Autodesk Inventor part; units mm, degrees
(part 2 of 3)
  spline S67 degree 3 poles (13.389509, -18.082427) (13.389509, -18.082427) (13.389509, -18.082427) (13.389509, -18.082427) (13.389509, -18.082427) (13.389509, -18.082427) (13.389509, -18.082427) (13.389509, -18.082427) (13.389509, -18.082427) (13.389509, -18.082427) (13.389509, -18.082427) (13.389509, -18.082427) (13.389509, -18.082427) (13.389509, -18.082427) (13.389509, -18.082427) (13.389449, -18.0824) (13.38145, -18.07871) (13.356188, -18.066962) (13.343085, -18.060852) (13.309671, -18.045163) (13.288775, -18.035295) (13.232029, -18.008233) (13.193942, -17.989858) (13.106898, -17.947135) (13.057393, -17.922403) (13.008015, -17.897214) knots 0 0 0 0 0.00003245 0.00003245 0.0000697 0.0000697 0.00012943 0.00012943 0.00021582 0.00021582 0.0003445 0.0003445 0.00053795 0.00053795 0.00077231 0.00077231 0.2100469 0.2100469 0.34914837 0.34914837 0.50737768 0.50737768 0.73605088 0.73605088 1 1 1 1
  arc A96 (13.389509, -18.082427) -> (14.254505, -17.40868) centre (0.000012, -0.000078) ccw
  arc A97 (13.008015, -17.897214) -> (14.168315, -16.993453) centre (0.000012, -0.000078) ccw
  arc A98 (13.008015, -17.897214) -> (14.168315, -16.993453) centre (0.000012, -0.000078) ccw
  spline S68 degree 3 poles (13.008015, -17.897214) (12.958136, -17.87177) (12.820927, -17.80036) (12.598988, -17.678088) (12.344986, -17.525914) (12.096924, -17.364239) (11.855202, -17.193219) (11.620622, -17.01253) (11.392126, -16.824355) (11.190356, -16.632755) (11.076365, -16.494814) (11.025839, -16.432401) knots 0 0 0 0 0.06771151 0.18704119 0.30636988 0.42569807 0.54502619 0.66435448 0.78368001 0.9029743 1 1 1 1
  spline S69 degree 3 poles (9.627578, -17.288804) (9.660216, -17.362174) (9.731294, -17.526398) (9.810284, -17.793198) (9.874079, -18.082249) (9.928439, -18.373318) (9.970943, -18.666356) (10.002239, -18.960794) (10.022375, -19.256206) (10.030442, -19.50947) (10.031705, -19.664143) (10.031705, -19.720138) knots 0 0 0 0 0.0970257 0.21631999 0.33564552 0.45497381 0.57430193 0.69363012 0.81295881 0.93228849 1 1 1 1
  spline S70 degree 3 poles (10.031705, -19.720138) (10.031705, -19.751925) (10.031556, -19.783696) (10.030978, -19.847374) (10.030538, -19.879187) (10.029238, -19.951858) (10.028283, -19.991171) (10.026684, -20.047685) (10.02605, -20.067721) (10.024929, -20.101167) (10.024444, -20.11462) (10.023769, -20.132892) (10.023548, -20.13864) (10.023433, -20.141656) (10.023401, -20.142482) (10.023369, -20.143307) (10.023337, -20.144133) knots 0 0 0 0 0.15652251 0.15652251 0.32009373 0.32009373 0.5482425 0.5482425 0.69838233 0.69838233 0.84400588 0.84400588 0.96648092 0.96648092 0.96648092 1 1 1 1
  arc A99 (9.030105, -20.608508) -> (10.023337, -20.144133) centre (0.000012, -0.000078) ccw
  arc A100 (8.69939, -20.343048) -> (10.031705, -19.720138) centre (0.000012, -0.000078) ccw
  arc A101 (8.69939, -20.343048) -> (10.031705, -19.720138) centre (0.000012, -0.000078) ccw
  spline S71 degree 3 poles (9.030105, -20.608508) (9.029452, -20.608004) (9.028799, -20.6075) (9.028146, -20.606995) (9.025218, -20.604734) (9.019043, -20.599964) (9.00106, -20.586016) (8.989646, -20.577144) (8.960561, -20.554413) (8.942385, -20.540143) (8.893084, -20.501131) (8.86004, -20.474743) (8.784685, -20.413721) (8.741925, -20.378593) (8.69939, -20.343048) knots 0 0 0 0 0.03353482 0.03353482 0.03353482 0.18383321 0.18383321 0.32755059 0.32755059 0.49103057 0.49103057 0.72729202 0.72729202 1 1 1 1
  arc A102 (7.092863, -18.473885) -> (6.374109, -18.179512) centre (6.56767, -18.731562) ccw
  spline S72 degree 3 poles (8.69939, -20.343048) (8.656423, -20.307143) (8.538545, -20.206992) (8.349378, -20.038399) (8.135606, -19.833519) (7.92974, -19.6207) (7.732134, -19.400179) (7.543642, -19.171822) (7.362748, -18.937519) (7.208672, -18.705825) (7.128233, -18.545977) (7.092863, -18.473885) knots 0 0 0 0 0.06771151 0.18704119 0.30636988 0.42569807 0.54502619 0.66435448 0.78368001 0.9029743 1 1 1 1
  arc A103 (5.932935, -18.328236) -> (6.374109, -18.179512) centre (0.000012, -0.000078) ccw
  arc A104 (5.932935, -18.328236) -> (5.539091, -18.997675) centre (6.113099, -18.884802) ccw
  spline S73 degree 3 poles (1.172852, -19.753927) (1.170424, -19.834191) (1.163209, -20.012992) (1.118616, -20.287643) (1.050679, -20.575748) (0.973366, -20.861578) (0.884515, -21.144038) (0.784961, -21.422896) (0.674928, -21.69779) (0.57231, -21.929473) (0.506337, -22.069377) (0.482042, -22.119826) knots 0 0 0 0 0.0970257 0.21631999 0.33564552 0.45497381 0.57430193 0.69363012 0.81295881 0.93228849 1 1 1 1
  arc A105 (1.705785, -19.18891) -> (1.172852, -19.753927) centre (1.757584, -19.771613) ccw
  arc A106 (1.705785, -19.18891) -> (2.168992, -19.142086) centre (0.000012, -0.000078) ccw
  arc A107 (2.804221, -19.589016) -> (2.168992, -19.142086) centre (2.234857, -19.723366) ccw
  spline S74 degree 3 poles (3.954541, -21.768801) (3.920641, -21.724235) (3.828004, -21.600365) (3.681096, -21.393906) (3.518274, -21.146594) (3.364926, -20.8933) (3.221345, -20.634337) (3.088393, -20.369761) (2.964172, -20.101081) (2.865515, -19.840911) (2.822663, -19.667171) (2.804221, -19.589016) knots 0 0 0 0 0.06771151 0.18704119 0.30636988 0.42569807 0.54502619 0.66435448 0.78368001 0.9029743 1 1 1 1
  arc A108 (3.954541, -21.768801) -> (5.392063, -21.457976) centre (0.000012, -0.000078) ccw
  spline S75 degree 3 poles (5.539091, -18.997675) (5.554585, -19.076467) (5.587338, -19.252391) (5.604978, -19.530079) (5.602854, -19.826078) (5.591082, -20.121946) (5.567313, -20.417094) (5.532306, -20.711114) (5.486201, -21.003601) (5.43771, -21.252309) (5.404523, -21.403386) (5.392063, -21.457976) knots 0 0 0 0 0.0970257 0.21631999 0.33564552 0.45497381 0.57430193 0.69363012 0.81295881 0.93228849 1 1 1 1
  spline S76 degree 3 poles (5.392063, -21.457976) (5.38499, -21.488967) (5.377775, -21.519907) (5.363042, -21.581861) (5.355533, -21.612778) (5.338095, -21.683338) (5.328417, -21.721453) (5.314282, -21.776194) (5.309205, -21.795587) (5.30067, -21.827945) (5.297204, -21.840952) (5.291318, -21.86296) (5.289572, -21.869423) (5.289558, -21.869479) (5.289558, -21.869479) (5.289558, -21.869479) (5.289558, -21.869479) (5.289558, -21.869479) (5.289558, -21.869479) (5.289558, -21.869479) (5.289558, -21.869479) (5.289558, -21.869479) (5.289558, -21.869479) (5.289558, -21.869479) (5.289558, -21.869479) (5.289558, -21.869479) (5.289558, -21.869479) (5.289558, -21.869479) knots 0 0 0 0 0.15149146 0.15149146 0.30980507 0.30980507 0.53062052 0.53062052 0.67593445 0.67593445 0.81687728 0.81687728 0.99922753 0.99922753 0.99946194 0.99946194 0.99965543 0.99965543 0.99978413 0.99978413 0.99987055 0.99987055 0.99993028 0.99993028 0.99996754 0.99996754 1 1 1 1
  arc A109 (4.217895, -22.101197) -> (5.289558, -21.869479) centre (0.000012, -0.000078) ccw
  arc A110 (3.954541, -21.768801) -> (5.392063, -21.457976) centre (0.000012, -0.000078) ccw
  spline S77 degree 3 poles (4.217895, -22.101197) (4.21737, -22.10056) (4.216846, -22.099923) (4.216321, -22.099286) (4.213971, -22.09643) (4.209012, -22.090405) (4.194583, -22.072805) (4.185429, -22.061615) (4.162132, -22.032982) (4.147586, -22.015025) (4.108202, -21.966022) (4.081859, -21.932942) (4.021972, -21.856682) (3.9881, -21.81292) (3.954541, -21.768801) knots 0 0 0 0 0.03353326 0.03353326 0.03353326 0.18383441 0.18383441 0.32755159 0.32755159 0.49103132 0.49103132 0.72729243 0.72729243 1 1 1 1
  spline S78 degree 3 poles (-0.988604, -22.102979) (-1.011737, -22.051987) (-1.074487, -21.910609) (-1.171771, -21.676636) (-1.275479, -21.399293) (-1.368619, -21.118227) (-1.450975, -20.833807) (-1.52172, -20.54628) (-1.58304, -20.256694) (-1.62133, -19.981094) (-1.624447, -19.802175) (-1.625035, -19.721876) knots 0 0 0 0 0.06771151 0.18704119 0.30636988 0.42569807 0.54502619 0.66435448 0.78368001 0.9029743 1 1 1 1
  arc A111 (-1.625035, -19.721876) -> (-2.144886, -19.144799) centre (-2.21002, -19.726162) ccw
  arc A112 (-2.606899, -19.087376) -> (-2.144886, -19.144799) centre (0.000012, -0.000078) ccw
  spline S79 degree 3 poles (-4.452151, -21.6725) (-4.47197, -21.697352) (-4.491895, -21.722098) (-4.53205, -21.771524) (-4.552229, -21.796121) (-4.598555, -21.852128) (-4.623812, -21.882269) (-4.660299, -21.925456) (-4.673287, -21.940726) (-4.695016, -21.966176) (-4.703783, -21.976391) (-4.718635, -21.993666) (-4.723012, -21.998732) (-4.72305, -21.998775) (-4.72305, -21.998775) (-4.72305, -21.998775) (-4.72305, -21.998775) (-4.72305, -21.998775) (-4.72305, -21.998775) (-4.72305, -21.998775) (-4.72305, -21.998775) (-4.72305, -21.998775) (-4.72305, -21.998775) (-4.72305, -21.998775) (-4.72305, -21.998775) (-4.72305, -21.998775) (-4.72305, -21.998775) (-4.72305, -21.998775) knots 0 0 0 0 0.15149146 0.15149146 0.30980507 0.30980507 0.53062052 0.53062052 0.67593445 0.67593445 0.81687728 0.81687728 0.99922753 0.99922753 0.99946194 0.99946194 0.99965543 0.99965543 0.99978413 0.99978413 0.99987055 0.99987055 0.99993028 0.99993028 0.99996754 0.99996754 1 1 1 1
  spline S80 degree 3 poles (-3.252199, -19.519638) (-3.272426, -19.59735) (-3.319247, -19.770062) (-3.423838, -20.027904) (-3.554181, -20.293668) (-3.693159, -20.555129) (-3.842635, -20.810735) (-4.001745, -21.060449) (-4.170189, -21.303966) (-4.321789, -21.507006) (-4.417239, -21.628722) (-4.452151, -21.6725) knots 0 0 0 0 0.0970257 0.21631999 0.33564552 0.45497381 0.57430193 0.69363012 0.81295881 0.93228849 1 1 1 1
  arc A113 (-5.789123, -21.742569) -> (-4.72305, -21.998775) centre (0.000012, -0.000078) ccw
  spline S81 degree 3 poles (-5.789123, -21.742569) (-5.789123, -21.742569) (-5.789123, -21.742569) (-5.789123, -21.742569) (-5.789123, -21.742569) (-5.789123, -21.742569) (-5.789123, -21.742569) (-5.789123, -21.742569) (-5.789123, -21.742569) (-5.789123, -21.742569) (-5.789123, -21.742569) (-5.789123, -21.742569) (-5.789123, -21.742568) (-5.789123, -21.742568) (-5.789123, -21.742568) (-5.789139, -21.742505) (-5.791242, -21.73395) (-5.797808, -21.706874) (-5.8012, -21.69282) (-5.809767, -21.656915) (-5.815081, -21.634425) (-5.829303, -21.573186) (-5.838684, -21.531952) (-5.859553, -21.437261) (-5.871082, -21.383136) (-5.882175, -21.328826) knots 0 0 0 0 0.00003245 0.00003245 0.0000697 0.0000697 0.00012943 0.00012943 0.00021582 0.00021582 0.0003445 0.0003445 0.00053795 0.00053795 0.00077231 0.00077231 0.2100469 0.2100469 0.34914836 0.34914836 0.50737768 0.50737768 0.73605088 0.73605088 1 1 1 1
  arc A114 (-5.882175, -21.328826) -> (-4.452151, -21.6725) centre (0.000012, -0.000078) ccw
  arc A115 (-5.882175, -21.328826) -> (-4.452151, -21.6725) centre (0.000012, -0.000078) ccw
  spline S82 degree 3 poles (-5.882175, -21.328826) (-5.893381, -21.273964) (-5.923099, -21.122167) (-5.96588, -20.872413) (-6.005273, -20.578947) (-6.033535, -20.284202) (-6.050537, -19.988587) (-6.055528, -19.692527) (-6.050871, -19.396557) (-6.026874, -19.119346) (-5.990099, -18.944219) (-5.972805, -18.865802) knots 0 0 0 0 0.06771151 0.18704119 0.30636988 0.42569807 0.54502619 0.66435448 0.78368001 0.9029743 1 1 1 1
  arc A116 (-5.972805, -18.865802) -> (-6.35121, -18.187517) centre (-6.544076, -18.73981) ccw
  arc A117 (-6.788862, -18.028726) -> (-6.35121, -18.187517) centre (0.000012, -0.000078) ccw
  arc A118 (-6.788862, -18.028726) -> (-7.51417, -18.306557) centre (-6.995018, -18.576197) ccw
  arc A119 (-2.606899, -19.087376) -> (-3.252199, -19.519638) centre (-2.686062, -19.666995) ccw
  arc A120 (-10.021072, -17.063722) -> (-10.239058, -16.31824) centre (-10.549985, -16.813769) ccw
  arc A121 (-10.630402, -16.066043) -> (-10.239058, -16.31824) centre (0.000012, -0.000078) ccw
  arc A122 (-10.630402, -16.066043) -> (-11.399348, -16.175512) centre (-10.953213, -16.553914) ccw
  spline S83 degree 3 poles (-13.41456, -17.594534) (-13.443199, -17.608326) (-13.471888, -17.621976) (-13.529511, -17.649085) (-13.558364, -17.662491) (-13.624403, -17.692851) (-13.660237, -17.709048) (-13.711849, -17.732128) (-13.730175, -17.74025) (-13.760795, -17.753752) (-13.773126, -17.759151) (-13.794003, -17.768271) (-13.800144, -17.770937) (-13.800196, -17.770959) (-13.800196, -17.770959) (-13.800197, -17.770959) (-13.800197, -17.770959) (-13.800197, -17.770959) (-13.800197, -17.770959) (-13.800197, -17.770959) (-13.800197, -17.770959) (-13.800197, -17.770959) (-13.800197, -17.770959) (-13.800197, -17.770959) (-13.800197, -17.770959) (-13.800197, -17.770959) (-13.800197, -17.770959) (-13.800197, -17.770959) knots 0 0 0 0 0.15149146 0.15149146 0.30980507 0.30980507 0.53062052 0.53062052 0.67593445 0.67593445 0.81687728 0.81687728 0.99922753 0.99922753 0.99946194 0.99946194 0.99965543 0.99965543 0.99978413 0.99978413 0.99987055 0.99987055 0.99993028 0.99993028 0.99996754 0.99996754 1 1 1 1
  spline S84 degree 3 poles (-11.399348, -16.175512) (-11.451291, -16.236752) (-11.568412, -16.372046) (-11.774518, -16.558973) (-12.007264, -16.741865) (-12.245922, -16.917132) (-12.491499, -17.08257) (-12.743199, -17.238519) (-13.00062, -17.384836) (-13.225302, -17.501991) (-13.364111, -17.570239) (-13.41456, -17.594534) knots 0 0 0 0 0.0970257 0.21631999 0.33564552 0.45497381 0.57430193 0.69363012 0.81295881 0.93228849 1 1 1 1
  arc A123 (-14.649532, -17.077573) -> (-13.800197, -17.770959) centre (0.000012, -0.000078) ccw
  arc A124 (-14.553853, -16.66443) -> (-13.41456, -17.594534) centre (0.000012, -0.000078) ccw
  arc A125 (-14.553853, -16.66443) -> (-13.41456, -17.594534) centre (0.000012, -0.000078) ccw
  spline S85 degree 3 poles (-14.649532, -17.077573) (-14.649361, -17.076766) (-14.64919, -17.075959) (-14.649019, -17.075152) (-14.648252, -17.071533) (-14.646633, -17.0639) (-14.641869, -17.041646) (-14.638828, -17.027512) (-14.630967, -16.991445) (-14.625997, -16.968877) (-14.61224, -16.907532) (-14.602802, -16.866311) (-14.580518, -16.771942) (-14.567422, -16.718175) (-14.553853, -16.66443) knots 0 0 0 0 0.0335333 0.0335333 0.0335333 0.18383438 0.18383438 0.32755156 0.32755156 0.4910313 0.4910313 0.72729242 0.72729242 1 1 1 1
  arc A126 (-13.566841, -14.406) -> (-13.613476, -13.630702) centre (-14.026873, -14.044619) ccw
  spline S86 degree 3 poles (-14.553853, -16.66443) (-14.540146, -16.61014) (-14.501058, -16.460481) (-14.431238, -16.216898) (-14.339399, -15.935403) (-14.236978, -15.657585) (-14.124033, -15.383867) (-14.000074, -15.114961) (-13.867462, -14.850322) (-13.725564, -14.610975) (-13.616447, -14.469147) (-13.566841, -14.406) knots 0 0 0 0 0.06771151 0.18704119 0.30636988 0.42569807 0.54502619 0.66435448 0.78368001 0.9029743 1 1 1 1
  arc A127 (-13.938889, -13.297747) -> (-13.613476, -13.630702) centre (0.000012, -0.000078) ccw
  arc A128 (-13.938889, -13.297747) -> (-14.712915, -13.233364) centre (-14.362168, -13.701553) ccw
  spline S87 degree 3 poles (-14.712915, -13.233364) (-14.777182, -13.28151) (-14.921473, -13.38735) (-15.164007, -13.523727) (-15.431615, -13.650243) (-15.70329, -13.768009) (-15.979523, -13.874654) (-16.259614, -13.970684) (-16.54314, -14.056051) (-16.788258, -14.120272) (-16.938773, -14.155921) (-16.993363, -14.168381) knots 0 0 0 0 0.0970257 0.21631999 0.33564552 0.45497381 0.57430193 0.69363012 0.81295881 0.93228849 1 1 1 1
  arc A129 (-16.548421, -9.862649) -> (-17.288715, -9.627643) centre (-17.050943, -10.162143) ccw
  arc A130 (-16.548421, -9.862649) -> (-16.305256, -10.259668) centre (0.000012, -0.000078) ccw
  arc A131 (-16.432311, -11.025905) -> (-16.305256, -10.259668) centre (-16.800394, -10.571218) ccw
  spline S88 degree 3 poles (-18.082338, -13.389575) (-18.081991, -13.388826) (-18.081645, -13.388077) (-18.081298, -13.387328) (-18.079745, -13.383971) (-18.076469, -13.376889) (-18.066872, -13.356253) (-18.060762, -13.34315) (-18.045073, -13.309737) (-18.035206, -13.288841) (-18.008143, -13.232095) (-17.989769, -13.194008) (-17.947045, -13.106963) (-17.922313, -13.057459) (-17.897124, -13.008081) knots 0 0 0 0 0.03353404 0.03353404 0.03353404 0.18383381 0.18383381 0.32755109 0.32755109 0.49103094 0.49103094 0.72729223 0.72729223 1 1 1 1
  arc A132 (-18.082338, -13.389575) -> (-17.40859, -14.254571) centre (0.000012, -0.000078) ccw
  arc A133 (-18.082338, -13.389575) -> (-17.40859, -14.254571) centre (0.000012, -0.000078) ccw
  arc A134 (-17.897124, -13.008081) -> (-16.993363, -14.168381) centre (0.000012, -0.000078) ccw
  arc A135 (-17.897124, -13.008081) -> (-16.993363, -14.168381) centre (0.000012, -0.000078) ccw
  spline S89 degree 3 poles (-16.993363, -14.168381) (-17.024354, -14.175454) (-17.055361, -14.182379) (-17.117571, -14.195985) (-17.148684, -14.202635) (-17.219823, -14.217539) (-17.258362, -14.225356) (-17.313816, -14.236372) (-17.333491, -14.240213) (-17.366347, -14.246562) (-17.379571, -14.249083) (-17.401953, -14.253329) (-17.408533, -14.25456) (-17.40859, -14.254571) (-17.40859, -14.254571) (-17.40859, -14.254571) (-17.40859, -14.254571) (-17.40859, -14.254571) (-17.40859, -14.254571) (-17.40859, -14.254571) (-17.40859, -14.254571) (-17.40859, -14.254571) (-17.40859, -14.254571) (-17.40859, -14.254571) (-17.40859, -14.254571) (-17.40859, -14.254571) (-17.40859, -14.254571) (-17.40859, -14.254571) knots 0 0 0 0 0.15149146 0.15149146 0.30980507 0.30980507 0.53062052 0.53062052 0.67593445 0.67593445 0.81687728 0.81687728 0.99922753 0.99922753 0.99946194 0.99946194 0.99965543 0.99965543 0.99978414 0.99978414 0.99987055 0.99987055 0.99993029 0.99993029 0.99996754 0.99996754 1 1 1 1
  spline S90 degree 3 poles (-17.897124, -13.008081) (-17.87168, -12.958201) (-17.80027, -12.820993) (-17.677999, -12.599054) (-17.525824, -12.345052) (-17.36415, -12.09699) (-17.193129, -11.855268) (-17.012441, -11.620687) (-16.824265, -11.392192) (-16.632666, -11.190422) (-16.494725, -11.07643) (-16.432311, -11.025905) knots 0 0 0 0 0.06771151 0.18704119 0.30636988 0.42569807 0.54502619 0.66435448 0.78368001 0.9029743 1 1 1 1
  spline S91 degree 3 poles (-18.997585, -5.539157) (-19.076378, -5.55465) (-19.252301, -5.587403) (-19.529989, -5.605044) (-19.825988, -5.602919) (-20.121856, -5.591148) (-20.417004, -5.567379) (-20.711024, -5.532372) (-21.003511, -5.486267) (-21.25222, -5.437776) (-21.403296, -5.404589) (-21.457887, -5.392129) knots 0 0 0 0 0.0970257 0.21631999 0.33564552 0.45497381 0.57430193 0.69363012 0.81295881 0.93228849 1 1 1 1
  spline S92 degree 3 poles (-17.288715, -9.627643) (-17.362084, -9.660282) (-17.526309, -9.73136) (-17.793109, -9.81035) (-18.082159, -9.874144) (-18.373228, -9.928505) (-18.666266, -9.971008) (-18.960704, -10.002305) (-19.256117, -10.02244) (-19.50938, -10.030508) (-19.664054, -10.03177) (-19.720048, -10.03177) knots 0 0 0 0 0.0970257 0.21631999 0.33564552 0.45497381 0.57430193 0.69363012 0.81295881 0.93228849 1 1 1 1
  spline S93 degree 3 poles (-19.720048, -10.03177) (-19.751835, -10.03177) (-19.783606, -10.031621) (-19.847284, -10.031044) (-19.879097, -10.030603) (-19.951769, -10.029304) (-19.991081, -10.028349) (-20.047596, -10.02675) (-20.067632, -10.026116) (-20.101078, -10.024995) (-20.11453, -10.02451) (-20.137296, -10.023668) (-20.143986, -10.023405) (-20.144043, -10.023403) (-20.144043, -10.023403) (-20.144043, -10.023403) (-20.144043, -10.023403) (-20.144043, -10.023403) (-20.144043, -10.023403) (-20.144043, -10.023403) (-20.144043, -10.023403) (-20.144043, -10.023403) (-20.144043, -10.023403) (-20.144043, -10.023403) (-20.144043, -10.023403) (-20.144043, -10.023403) (-20.144043, -10.023403) (-20.144043, -10.023403) knots 0 0 0 0 0.15149146 0.15149146 0.30980507 0.30980507 0.53062052 0.53062052 0.67593445 0.67593445 0.81687728 0.81687728 0.99922753 0.99922753 0.99946194 0.99946194 0.99965543 0.99965543 0.99978413 0.99978413 0.99987055 0.99987055 0.99993028 0.99993028 0.99996754 0.99996754 1 1 1 1
  arc A136 (-20.608419, -9.030171) -> (-20.144043, -10.023403) centre (0.000012, -0.000078) ccw
  arc A137 (-20.342959, -8.699455) -> (-19.720048, -10.03177) centre (0.000012, -0.000078) ccw
  arc A138 (-20.342959, -8.699455) -> (-19.720048, -10.03177) centre (0.000012, -0.000078) ccw
  arc A139 (-18.473796, -7.092928) -> (-18.179423, -6.374175) centre (-18.731473, -6.567735) ccw
  spline S94 degree 3 poles (-20.342959, -8.699455) (-20.307053, -8.656489) (-20.206902, -8.53861) (-20.03831, -8.349443) (-19.83343, -8.135672) (-19.62061, -7.929806) (-19.400089, -7.7322) (-19.171732, -7.543707) (-18.93743, -7.362814) (-18.705736, -7.208737) (-18.545887, -7.128299) (-18.473796, -7.092928) knots 0 0 0 0 0.06771151 0.18704119 0.30636988 0.42569807 0.54502619 0.66435448 0.78368001 0.9029743 1 1 1 1
  arc A140 (-18.328146, -5.933001) -> (-18.179423, -6.374175) centre (0.000012, -0.000078) ccw
  arc A141 (-18.328146, -5.933001) -> (-18.997585, -5.539157) centre (-18.884713, -6.113164) ccw
  spline S95 degree 3 poles (-20.608419, -9.030171) (-20.608419, -9.030171) (-20.608419, -9.030171) (-20.608419, -9.030171) (-20.608419, -9.030171) (-20.608419, -9.030171) (-20.608419, -9.030171) (-20.608419, -9.030171) (-20.608419, -9.030171) (-20.608419, -9.030171) (-20.608419, -9.030171) (-20.608419, -9.030171) (-20.608419, -9.030171) (-20.608419, -9.030171) (-20.608419, -9.030171) (-20.608378, -9.030119) (-20.603002, -9.023141) (-20.585926, -9.001126) (-20.577054, -8.989711) (-20.554323, -8.960627) (-20.540053, -8.94245) (-20.501042, -8.893149) (-20.474653, -8.860105) (-20.413631, -8.78475) (-20.378503, -8.74199) (-20.342959, -8.699455) knots 0 0 0 0 0.00003245 0.00003245 0.0000697 0.0000697 0.00012942 0.00012942 0.00021582 0.00021582 0.0003445 0.0003445 0.00053794 0.00053794 0.00077231 0.00077231 0.2100469 0.2100469 0.34914836 0.34914836 0.50737768 0.50737768 0.73605088 0.73605088 1 1 1 1
  arc A142 (-19.188821, -1.705851) -> (-19.141996, -2.169058) centre (0.000012, -0.000078) ccw
  arc A143 (-19.188821, -1.705851) -> (-19.753837, -1.172917) centre (-19.771523, -1.75765) ccw
  spline S96 degree 3 poles (-22.119736, -0.482107) (-22.148376, -0.468315) (-22.176935, -0.454396) (-22.234057, -0.426247) (-22.262528, -0.412047) (-22.327439, -0.379345) (-22.362445, -0.361428) (-22.412668, -0.335466) (-22.430445, -0.326201) (-22.460092, -0.31068) (-22.472002, -0.304406) (-22.492149, -0.29377) (-22.498061, -0.290631) (-22.498112, -0.290604) (-22.498112, -0.290604) (-22.498112, -0.290604) (-22.498112, -0.290604) (-22.498112, -0.290604) (-22.498112, -0.290604) (-22.498112, -0.290604) (-22.498112, -0.290604) (-22.498112, -0.290604) (-22.498112, -0.290604) (-22.498112, -0.290604) (-22.498112, -0.290604) (-22.498112, -0.290604) (-22.498112, -0.290604) (-22.498112, -0.290604) knots 0 0 0 0 0.15149146 0.15149146 0.30980507 0.30980507 0.53062052 0.53062052 0.67593445 0.67593445 0.81687728 0.81687728 0.99922753 0.99922753 0.99946194 0.99946194 0.99965543 0.99965543 0.99978413 0.99978413 0.99987055 0.99987055 0.99993028 0.99993028 0.99996754 0.99996754 1 1 1 1
  spline S97 degree 3 poles (-19.753837, -1.172917) (-19.834101, -1.17049) (-20.012902, -1.163275) (-20.287553, -1.118681) (-20.575658, -1.050744) (-20.861489, -0.973431) (-21.143948, -0.884581) (-21.422807, -0.785027) (-21.697701, -0.674993) (-21.929384, -0.572375) (-22.069287, -0.506402) (-22.119736, -0.482107) knots 0 0 0 0 0.0970257 0.21631999 0.33564552 0.45497381 0.57430193 0.69363012 0.81295881 0.93228849 1 1 1 1
  arc A144 (-22.485553, 0.805753) -> (-22.498112, -0.290604) centre (0.000012, -0.000078) ccw
  spline S98 degree 3 poles (-22.485553, 0.805753) (-22.484815, 0.806122) (-22.484078, 0.806492) (-22.48334, 0.806861) (-22.480033, 0.808517) (-22.473056, 0.812011) (-22.452686, 0.822162) (-22.439739, 0.828597) (-22.40664, 0.844938) (-22.385897, 0.855123) (-22.329358, 0.882616) (-22.291246, 0.900937) (-22.203572, 0.942354) (-22.15337, 0.965638) (-22.10289, 0.988538) knots 0 0 0 0 0.03353265 0.03353265 0.03353265 0.18383488 0.18383488 0.32755197 0.32755197 0.49103161 0.49103161 0.72729259 0.72729259 1 1 1 1
  arc A145 (-22.10289, 0.988538) -> (-22.119736, -0.482107) centre (0.000012, -0.000078) ccw
  arc A146 (-22.10289, 0.988538) -> (-22.119736, -0.482107) centre (0.000012, -0.000078) ccw
  spline S99 degree 3 poles (-22.10289, 0.988538) (-22.051897, 1.011671) (-21.910519, 1.074422) (-21.676546, 1.171706) (-21.399204, 1.275413) (-21.118138, 1.368553) (-20.833717, 1.45091) (-20.546191, 1.521655) (-20.256605, 1.582974) (-19.981004, 1.621264) (-19.802085, 1.624381) (-19.721786, 1.62497) knots 0 0 0 0 0.06771151 0.18704119 0.30636988 0.42569807 0.54502619 0.66435448 0.78368001 0.9029743 1 1 1 1
  arc A147 (-19.721786, 1.62497) -> (-19.14471, 2.14482) centre (-19.726073, 2.209954) ccw
  arc A148 (-19.087287, 2.606833) -> (-19.14471, 2.14482) centre (0.000012, -0.000078) ccw
  arc A149 (-19.087287, 2.606833) -> (-19.519548, 3.252133) centre (-19.666906, 2.685996) ccw
  spline S100 degree 3 poles (-19.519548, 3.252133) (-19.59726, 3.272361) (-19.769972, 3.319182) (-20.027814, 3.423772) (-20.293579, 3.554116) (-20.555039, 3.693093) (-20.810645, 3.842569) (-21.060359, 4.001679) (-21.303877, 4.170124) (-21.506916, 4.321723) (-21.628632, 4.417174) (-21.67241, 4.452085) knots 0 0 0 0 0.0970257 0.21631999 0.33564552 0.45497381 0.57430193 0.69363012 0.81295881 0.93228849 1 1 1 1
  arc A150 (-18.028636, 6.788796) -> (-18.187427, 6.351145) centre (0.000012, -0.000078) ccw
  arc A151 (-18.028636, 6.788796) -> (-18.306467, 7.514104) centre (-18.576107, 6.994952) ccw
  spline S101 degree 3 poles (-20.138338, 9.163028) (-20.158157, 9.18788) (-20.177849, 9.212812) (-20.2171, 9.262958) (-20.23659, 9.288105) (-20.280884, 9.345733) (-20.304649, 9.377063) (-20.338635, 9.422246) (-20.350631, 9.438305) (-20.370608, 9.465153) (-20.378616, 9.475974) (-20.392153, 9.494297) (-20.396118, 9.499691) (-20.396152, 9.499737) (-20.396152, 9.499738) (-20.396152, 9.499738) (-20.396152, 9.499738) (-20.396152, 9.499738) (-20.396152, 9.499738) (-20.396152, 9.499738) (-20.396152, 9.499738) (-20.396152, 9.499738) (-20.396152, 9.499738) (-20.396152, 9.499738) (-20.396152, 9.499738) (-20.396152, 9.499738) (-20.396152, 9.499738) (-20.396152, 9.499738) knots 0 0 0 0 0.15149146 0.15149146 0.30980507 0.30980507 0.53062052 0.53062052 0.67593445 0.67593445 0.81687728 0.81687728 0.99922753 0.99922753 0.99946194 0.99946194 0.99965543 0.99965543 0.99978413 0.99978413 0.99987055 0.99987055 0.99993028 0.99993028 0.99996754 0.99996754 1 1 1 1
  spline S102 degree 3 poles (-18.306467, 7.514104) (-18.377729, 7.551117) (-18.535693, 7.635196) (-18.763797, 7.79454) (-18.993894, 7.980753) (-19.217873, 8.174427) (-19.43381, 8.377033) (-19.641857, 8.58772) (-19.841787, 8.806129) (-20.006001, 8.999108) (-20.103426, 9.11925) (-20.138338, 9.163028) knots 0 0 0 0 0.0970257 0.21631999 0.33564552 0.45497381 0.57430193 0.69363012 0.81295881 0.93228849 1 1 1 1
  arc A152 (-19.909145, 10.482071) -> (-20.396152, 9.499738) centre (0.000012, -0.000078) ccw
  arc A153 (-19.48507, 10.480724) -> (-20.138338, 9.163028) centre (0.000012, -0.000078) ccw
  arc A154 (-19.48507, 10.480724) -> (-20.138338, 9.163028) centre (0.000012, -0.000078) ccw
  spline S103 degree 3 poles (-19.909145, 10.482071) (-19.90832, 10.482084) (-19.907495, 10.482097) (-19.90667, 10.48211) (-19.902972, 10.482167) (-19.89517, 10.482288) (-19.872414, 10.482595) (-19.857957, 10.482775) (-19.821046, 10.483137) (-19.797938, 10.483314) (-19.735069, 10.483552) (-19.692781, 10.483523) (-19.59582, 10.482797) (-19.540487, 10.481994) (-19.48507, 10.480724) knots 0 0 0 0 0.03353442 0.03353442 0.03353442 0.18383352 0.18383352 0.32755085 0.32755085 0.49103076 0.49103076 0.72729213 0.72729213 1 1 1 1
  spline S104 degree 3 poles (-19.48507, 10.480724) (-19.429091, 10.479441) (-19.274486, 10.474636) (-19.021474, 10.460769) (-18.7266, 10.433871) (-18.432957, 10.395838) (-18.140969, 10.346633) (-17.851222, 10.285619) (-17.563709, 10.215219) (-17.298788, 10.130139) (-17.136235, 10.055317) (-17.063633, 10.021007) knots 0 0 0 0 0.06771151 0.18704119 0.30636988 0.42569807 0.54502619 0.66435448 0.78368001 0.9029743 1 1 1 1
  arc A155 (-17.063633, 10.021007) -> (-16.31815, 10.238992) centre (-16.813679, 10.549919) ccw
  arc A156 (-16.065954, 10.630336) -> (-16.31815, 10.238992) centre (0.000012, -0.000078) ccw
  arc A157 (-16.065954, 10.630336) -> (-16.175423, 11.399283) centre (-16.553825, 10.953147) ccw
  arc A158 (-18.865712, 5.972739) -> (-18.187427, 6.351145) centre (-18.73972, 6.544011) ccw
  spline S105 degree 3 poles (-13.233274, 14.71285) (-13.28142, 14.777117) (-13.38726, 14.921407) (-13.523638, 15.163941) (-13.650153, 15.431549) (-13.767919, 15.703224) (-13.874564, 15.979457) (-13.970595, 16.259549) (-14.055961, 16.543074) (-14.120183, 16.788193) (-14.155832, 16.938707) (-14.168291, 16.993298) knots 0 0 0 0 0.0970257 0.21631999 0.33564552 0.45497381 0.57430193 0.69363012 0.81295881 0.93228849 1 1 1 1
  spline S106 degree 3 poles (-14.168291, 16.993298) (-14.175365, 17.024288) (-14.182289, 17.055295) (-14.195896, 17.117506) (-14.202545, 17.148619) (-14.217449, 17.219758) (-14.225266, 17.258297) (-14.236283, 17.31375) (-14.240123, 17.333425) (-14.246473, 17.366282) (-14.248993, 17.379505) (-14.253239, 17.401887) (-14.254471, 17.408468) (-14.254481, 17.408524) (-14.254481, 17.408524) (-14.254481, 17.408524) (-14.254481, 17.408524) (-14.254481, 17.408524) (-14.254481, 17.408524) (-14.254481, 17.408524) (-14.254481, 17.408524) (-14.254481, 17.408524) (-14.254481, 17.408524) (-14.254481, 17.408524) (-14.254481, 17.408524) (-14.254481, 17.408524) (-14.254481, 17.408524) (-14.254481, 17.408524) knots 0 0 0 0 0.15149146 0.15149146 0.30980507 0.30980507 0.53062052 0.53062052 0.67593445 0.67593445 0.81687728 0.81687728 0.99922753 0.99922753 0.99946195 0.99946195 0.99965543 0.99965543 0.99978414 0.99978414 0.99987055 0.99987055 0.99993029 0.99993029 0.99996754 0.99996754 1 1 1 1
  arc A159 (-13.389485, 18.082272) -> (-14.254481, 17.408524) centre (0.000012, -0.000078) ccw
  arc A160 (-13.007991, 17.897059) -> (-14.168291, 16.993298) centre (0.000012, -0.000078) ccw
  arc A161 (-13.007991, 17.897059) -> (-14.168291, 16.993298) centre (0.000012, -0.000078) ccw
  arc A162 (-11.025815, 16.432245) -> (-10.259578, 16.305191) centre (-10.571128, 16.800328) ccw
  arc A163 (-9.862559, 16.548356) -> (-10.259578, 16.305191) centre (0.000012, -0.000078) ccw
  spline S107 degree 3 poles (-13.007991, 17.897059) (-12.958112, 17.871614) (-12.820903, 17.800205) (-12.598964, 17.677933) (-12.344962, 17.525758) (-12.0969, 17.364084) (-11.855178, 17.193063) (-11.620598, 17.012375) (-11.392102, 16.8242) (-11.190332, 16.6326) (-11.076341, 16.494659) (-11.025815, 16.432245) knots 0 0 0 0 0.06771151 0.18704119 0.30636988 0.42569807 0.54502619 0.66435448 0.78368001 0.9029743 1 1 1 1
  arc A164 (-9.862559, 16.548356) -> (-9.627554, 17.288649) centre (-10.162053, 17.050878) ccw
  spline S108 degree 3 poles (-13.389485, 18.082272) (-13.389485, 18.082272) (-13.389485, 18.082272) (-13.389485, 18.082272) (-13.389485, 18.082272) (-13.389485, 18.082272) (-13.389485, 18.082272) (-13.389485, 18.082272) (-13.389485, 18.082272) (-13.389485, 18.082272) (-13.389485, 18.082272) (-13.389485, 18.082272) (-13.389485, 18.082272) (-13.389485, 18.082272) (-13.389485, 18.082272) (-13.389425, 18.082244) (-13.381426, 18.078555) (-13.356163, 18.066807) (-13.343061, 18.060697) (-13.309647, 18.045007) (-13.288751, 18.03514) (-13.232005, 18.008077) (-13.193918, 17.989703) (-13.106874, 17.946979) (-13.057369, 17.922247) (-13.007991, 17.897059) knots 0 0 0 0 0.00003245 0.00003245 0.0000697 0.0000697 0.00012943 0.00012943 0.00021582 0.00021582 0.0003445 0.0003445 0.00053795 0.00053795 0.00077231 0.00077231 0.21004691 0.21004691 0.34914837 0.34914837 0.50737768 0.50737768 0.73605088 0.73605088 1 1 1 1
  arc A165 (-13.297657, 13.938823) -> (-13.233274, 14.71285) centre (-13.701464, 14.362102) ccw
  arc A166 (-13.297657, 13.938823) -> (-13.630612, 13.61341) centre (0.000012, -0.000078) ccw
  arc A167 (-14.40591, 13.566775) -> (-13.630612, 13.61341) centre (-14.04453, 14.026807) ccw
  spline S109 degree 3 poles (-16.664341, 14.553787) (-16.61005, 14.54008) (-16.460391, 14.500993) (-16.216809, 14.431172) (-15.935313, 14.339334) (-15.657495, 14.236912) (-15.383777, 14.123968) (-15.114871, 14.000008) (-14.850232, 13.867396) (-14.610886, 13.725498) (-14.469057, 13.616381) (-14.40591, 13.566775) knots 0 0 0 0 0.06771151 0.18704119 0.30636988 0.42569807 0.54502619 0.66435448 0.78368001 0.9029743 1 1 1 1
  spline S110 degree 3 poles (-17.077496, 14.649544) (-17.077496, 14.649544) (-17.077496, 14.649544) (-17.077496, 14.649544) (-17.077496, 14.649544) (-17.077496, 14.649544) (-17.077496, 14.649544) (-17.077496, 14.649544) (-17.077496, 14.649544) (-17.077496, 14.649544) (-17.077496, 14.649544) (-17.077496, 14.649544) (-17.077496, 14.649544) (-17.077496, 14.649544) (-17.077495, 14.649544) (-17.077431, 14.64953) (-17.068811, 14.647712) (-17.041567, 14.641875) (-17.027433, 14.638831) (-16.991365, 14.630963) (-16.968796, 14.625989) (-16.907449, 14.61222) (-16.866227, 14.602774) (-16.771855, 14.580473) (-16.718087, 14.567367) (-16.664341, 14.553787) knots 0 0 0 0 0.00003245 0.00003245 0.0000697 0.0000697 0.00012943 0.00012943 0.00021582 0.00021582 0.0003445 0.0003445 0.00053795 0.00053795 0.00077231 0.00077231 0.2100469 0.2100469 0.34914836 0.34914836 0.50737768 0.50737768 0.73605088 0.73605088 1 1 1 1
  arc A168 (-17.077496, 14.649544) -> (-17.770882, 13.800209) centre (0, 0) ccw
  arc A169 (-16.664341, 14.553787) -> (-17.594444, 13.414494) centre (0.000012, -0.000078) ccw
  spline S111 degree 3 poles (-17.594444, 13.414494) (-17.608237, 13.443139) (-17.621889, 13.471834) (-17.648999, 13.529469) (-17.662406, 13.558328) (-17.692769, 13.62438) (-17.708967, 13.660221) (-17.732048, 13.711843) (-17.74017, 13.730173) (-17.753673, 13.760799) (-17.759073, 13.773133) (-17.766393, 13.789892) (-17.768689, 13.795167) (-17.769893, 13.797936) (-17.770223, 13.798693) (-17.770552, 13.799451) (-17.770882, 13.800209) knots 0 0 0 0 0.15652243 0.15652243 0.32009355 0.32009355 0.54824219 0.54824219 0.69838193 0.69838193 0.84400541 0.84400541 0.96648151 0.96648151 0.96648151 1 1 1 1
  spline S112 degree 3 poles (-16.175423, 11.399283) (-16.236662, 11.451225) (-16.371956, 11.568346) (-16.558883, 11.774453) (-16.741775, 12.007199) (-16.917042, 12.245857) (-17.082481, 12.491433) (-17.23843, 12.743133) (-17.384746, 13.000555) (-17.501902, 13.225237) (-17.570149, 13.364045) (-17.594444, 13.414494) knots 0 0 0 0 0.0970257 0.21631999 0.33564552 0.45497381 0.57430193 0.69363012 0.81295881 0.93228849 1 1 1 1
  arc A170 (-16.664341, 14.553787) -> (-17.594444, 13.414494) centre (0.000012, -0.000078) ccw
  circle A171 centre (0.000012, -0.000078) radius 3.5
  circle A172 centre (8, 0) radius 2.5
  circle A173 centre (2.47207, 7.608387) radius 2.5
  circle A174 centre (-6.47216, 4.702134) radius 2.5
  circle A175 centre (-6.472069, -4.702415) radius 2.5
  circle A176 centre (2.472218, -7.608494) radius 2.5
  dimension "d2" = 7
  dimension "d3" = 5
  dimension "d4" = 8
  dimension "d7" = 360
  constraints: 342 point on circle, 177 centre point, 4 coincident, 1 horizontal alignment, 237 other
  measures "d2" diameter of A171
  measures "d3" diameter of A172
  measures "d4" distance of A172.centre point (0, 0)